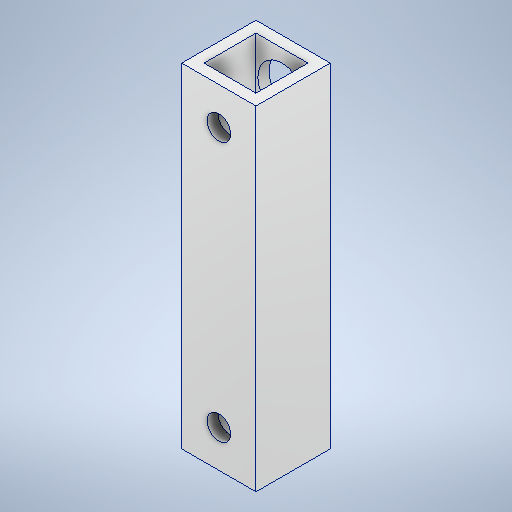
# Autodesk Inventor part: bearing_base
Saved by Autodesk Inventor 2025 (Build 290162000, 162)
## iProperties
Created: 2024-04-25
Part Number: bearing_base
Material: Hliník 6061
Document SubType Name: Modeling
Designer: rader
Density: 2.7 g/cm^3
Appearance: Hliník – plochý
Author: rader
Autodesk Inventor part; units mm, degrees
ref_plane "YZ Plane" through (0, 0, 0) normal (1, 0, 0) x (0, 1, 0)
ref_plane "XZ Plane" through (0, 0, 0) normal (0, 1, 0) x (-1, 0, 0)
ref_plane "XY Plane" through (0, 0, 0) normal (0, 0, 1) x (1, 0, 0)
sketch "Náčrt1" plane through (0, 0, 0) normal (0, 0, 1) x (1, 0, 0)
  line L0 (0, 7) -> (0, -7) projected
  line L1 (-7, 0) -> (7, 0) projected
  line L2 (-3.5, 3.5) -> (3.5, 3.5)
  line L3 (3.5, 3.5) -> (3.5, -3.5)
  line L4 (3.5, -3.5) -> (-3.5, -3.5)
  line L5 (-3.5, -3.5) -> (-3.5, 3.5)
  line L6 (-5, 5) -> (5, 5)
  line L7 (5, 5) -> (5, -5)
  line L8 (5, -5) -> (-5, -5)
  line L9 (-5, -5) -> (-5, 5)
  point P0 (0, 0)
  dimension "d1" = 10
  dimension "d2" = 10
  dimension "d3" = 1.5
  dimension "d4" = 1.5
  dimension "d5" = 1.5
  dimension "d6" = 1.5
  constraints: 16 end point, 4 parallel, 2 horizontal, 2 perpendicular, 2 other
  measures "d1" distance of L6.start L6.end
  measures "d2" distance of L6.end L7.end
  measures "d3" distance between parallel lines of L7 L3
  measures "d4" distance between parallel lines of L9 L5
  measures "d5" distance between parallel lines of L6 L2
  measures "d6" distance between parallel lines of L8 L4
extrude "Vysunutí1" add sketch "Náčrt1" along normal mid plane 22.5 contours L6 L7 L1 L3 L2 L0 | L0 L2 L5 L1 L9 L6 | L1 L5 L4 L0 L8 L9 | L7 L8 L0 L4 L3 L1
sketch "Náčrt2" plane through (-5, 5, 11.25) normal (0, 1, 0) x (1, 0, 0)
  line L0 (12, 11.25) -> (-2, 11.25) projected
  line L1 (5, 27) -> (5, -4.5) projected
  line L2 (10, 0) -> (0, 0) projected
  line L3 (0, 22.5) -> (0, 0) projected
  point P0 (5, 11.25)
  point P1 (5, 5)
  dimension "d10" = 5
  dimension "d11" = 5
  measures "d10" distance from line of L3 point (5, 5)
  measures "d11" distance from line of L2 point (5, 5)
hole "Díra1" at (0, 5, 6.25) direction (0, -1, 0) diameter 3.2 end through all counterbore diameter 6.5 counterbore depth 2
sketch "Náčrt3" plane through (-5, 5, 11.25) normal (0, 1, 0) x (1, 0, 0)
  line L0 (0, 22.5) -> (0, 0) projected
  line L1 (0, 22.5) -> (10, 22.5) projected
  point P0 (5, 11.25)
  point P1 (5, 15)
  point P2 (5, 3)
  dimension "d19" = 5
  dimension "d20" = 5
  dimension "d21" = 12
  dimension "d22" = 7.5
  measures "d19" distance from line of L0 point (5, 15)
  measures "d20" distance from line of L0 point (5, 3)
  measures "d21" distance of point (5, 15) point (5, 3)
  measures "d22" distance from line of L1 point (5, 15)
hole "Díra2" at (0, 5, -3.75) at (0, 5, 8.25) direction (0, -1, 0) diameter 2.459 depth 1.5 thread size "M3x0.5" class "6H" standard "ISO Metric profile"
mirror "Zrcadlit1" about plane through (0, 0, -11.25) normal (0, 0, -1) of "Vysunutí1", "Díra1", "Díra2"
